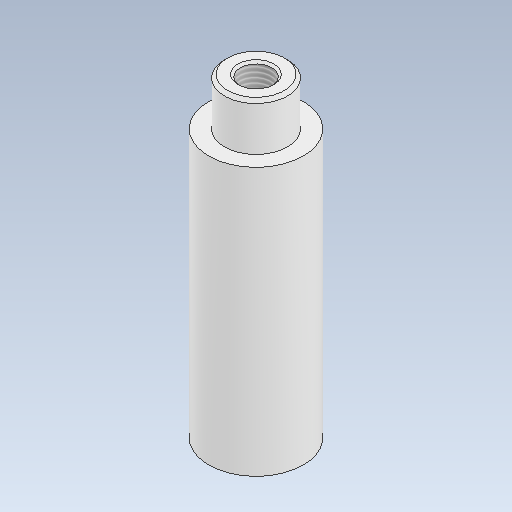
# Autodesk Inventor part: rączka_korby
Saved by Autodesk Inventor 2020 (Build 240168000, 168)
## iProperties
Created: 2020-08-09
Part Number: rączka_korby
Material: ABS Plastic
Document SubType Name: Modeling
Designer: Hesekiel
Density: 1.06 g/cm^3
Appearance: Smooth - White
Mass: 65.3123 g
Surface Area: 115.735 cm^2
Volume: 61.6153 cm^3
Author: Hesekiel
Autodesk Inventor part; units mm, degrees
ref_plane "YZ Plane" through (0, 0, 0) normal (1, 0, 0) x (0, 1, 0)
ref_plane "XZ Plane" through (0, 0, 0) normal (0, 1, 0) x (-1, 0, 0)
ref_plane "XY Plane" through (0, 0, 0) normal (0, 0, 1) x (1, 0, 0)
sketch "Sketch1" plane through (0, 0, 0) normal (0, 1, 0) x (-1, 0, 0)
  circle A0 centre (0, 0) radius 10
  dimension "d0" = 20
  constraints: 1 centre point, 1 coincident
  measures "d0" diameter of A0
extrude "Extrusion1" add sketch "Sketch1" along normal blind 100
sketch "Sketch2" plane through (0, 100, 0) normal (0, 1, 0) x (1, 0, 0)
  circle A0 centre (0, 0) radius 5
  dimension "d3" = 10
  constraints: 1 centre point, 1 coincident
  measures "d3" diameter of A0
extrude "Extrusion2" cut sketch "Sketch2" against normal blind 30
thread "Thread1" size "M10x1.5" class "6H" standard "ANSI Metric M Profile" full length
chamfer "Chamfer1" distance 1 angle 45 1 edges at (10, 100, 0)
chamfer "Chamfer2" distance 0.7 angle 45 1 edges at (-5, 100, 0)
sketch "Sketch8" plane through (0, 0, 0) normal (0, -1, 0) x (1, 0, 0)
  circle A0 centre (0, 0) radius 15
  dimension "d49" = 30
  constraints: 1 centre point, 1 coincident
  measures "d49" diameter of A0
extrude "Extrusion3" add sketch "Sketch8" against normal blind 85
sketch "Sketch9" plane through (0, 85, 0) normal (0, 1, 0) x (1, 0, 0)
  circle A0 centre (0, 0) radius 5 projected
extrude "Extrusion4" cut sketch "Sketch9" against normal blind 25
sketch "Sketch3" plane through (0, 70, 0) normal (0, 1, 0) x (1, 0, 0)
  point P0 (0, 0)
sketch "Sketch4" plane through (0, 70, 0) normal (0, 1, 0) x (1, 0, 0)
  point P0 (0, 0)
sketch "Sketch5" plane through (0, 70, 0) normal (0, 1, 0) x (1, 0, 0)
  point P0 (0, 0)
sketch "Sketch6" plane through (0, 70, 0) normal (0, 1, 0) x (1, 0, 0)
  point P0 (0, 0)
sketch "Sketch7" plane through (0, 70, 0) normal (0, 1, 0) x (1, 0, 0)
  point P0 (0, 0)
body "Solid1"
